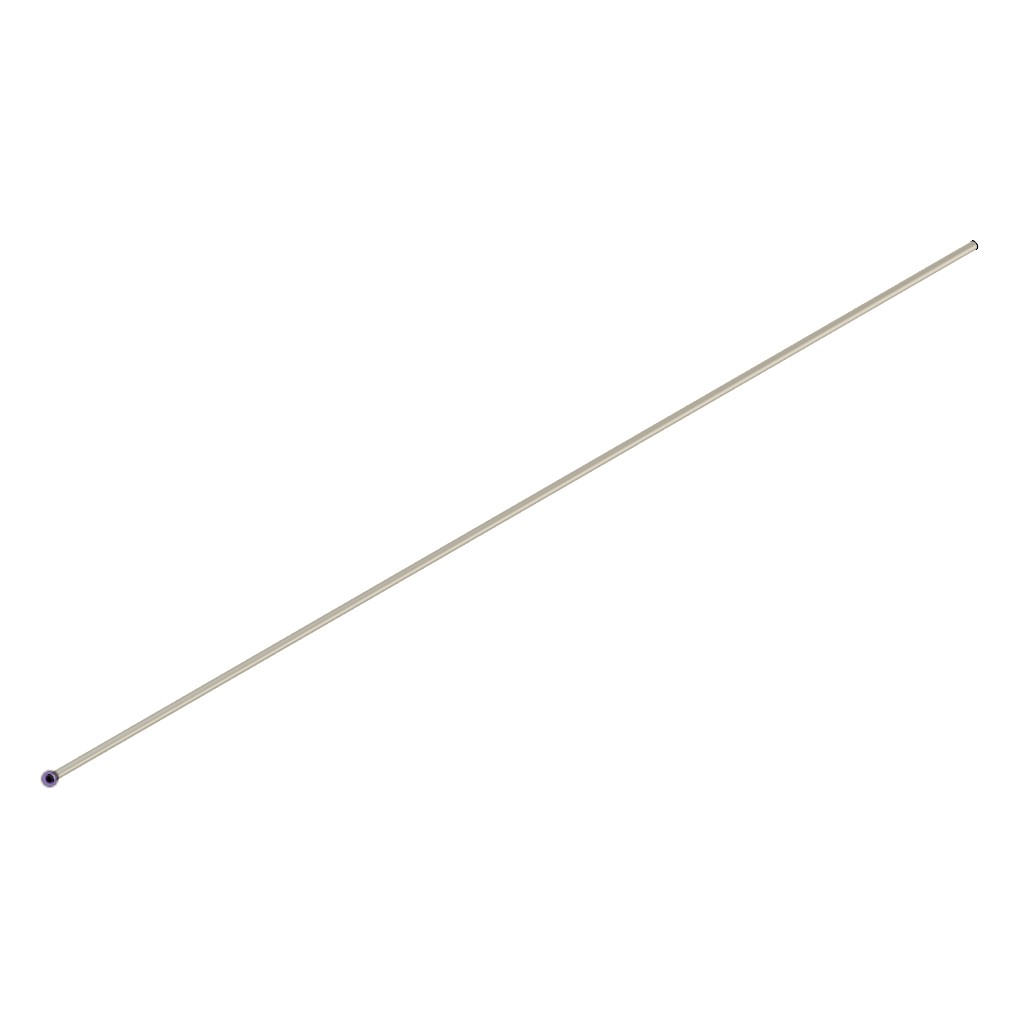
a3-1 (Autodesk Fusion 360 design; units mm, degrees)
part number: 2026-09-09-17-31-48-960
Autodesk Fusion 360 part; units mm, degrees
sketch "Sketch1" plane through (0, 0, 0) normal (0, 1, 0) x (1, 0, 0)
  circle A0 centre (0, 0) radius 7.1652
  dimension "d8" = 14.3304
  constraint coincident A0.centre origin
  measures "d8" diameter of A0
extrude "Extrude2" add sketch "Sketch1" along normal blind 1905
equation "Force = 300 lbforce"
equation "Elastic_Modulus = 10000000 psi"
equation "Deflection = 0.009 in"
equation "diameter = 0.5641895835 in"
equation "Length = Deflection * ( diameter ^ 2 * PI / 4 ) * Elastic_Modulus / Force"
equation "d8 = diameter"
equation "d9 = Length"
